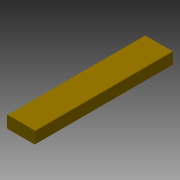
# Autodesk Inventor part: 2x4x17
Saved by Autodesk Inventor 2015 (Build 190159000, 159)
## iProperties
Created: 2015-01-03
Part Number: 2x4x17
Material: Wood (Oak)
Document SubType Name: Modeling
Designer: Peter
Mass: 3130.43 g
Surface Area: 3097.88 cm^2
Volume: 4118.99 cm^3
Density: 0.76 g/cm^3
Appearance: Gold
Author: Peter
Autodesk Inventor part; units mm, degrees
ref_plane "YZ Plane" through (0, 0, 0) normal (1, 0, 0) x (0, 1, 0)
ref_plane "XZ Plane" through (0, 0, 0) normal (0, 1, 0) x (-1, 0, 0)
ref_plane "XY Plane" through (0, 0, 0) normal (0, 0, 1) x (1, 0, 0)
sketch "Sketch1" plane through (0, 0, 0) normal (0, 0, 1) x (1, 0, 0)
  line L0 (0, 0) -> (88.9, 0)
  line L1 (88.9, 0) -> (88.9, 34.925)
  line L2 (85.725, 38.1) -> (3.175, 38.1)
  line L3 (0, 34.925) -> (0, 0)
  arc A0 (3.175, 38.1) -> (0, 34.925) centre (3.175, 34.925) ccw
  arc A1 (88.9, 34.925) -> (85.725, 38.1) centre (85.725, 34.925) ccw
  point P0 (88.9, 38.1)
  point P1 (0, 38.1)
  dimension "Width" = 88.9
  dimension "Height" = 38.1
  dimension "d2" = 3.175
  constraints: 8 end point, 4 point on circle, 4 point on line, 4 tangent, 2 centre point, 2 parallel, 1 equal radius, 1 horizontal, 1 perpendicular
  measures "Width" distance of point (88.9, 38.1) point (0, 38.1)
  measures "Height" distance of L0.end point (88.9, 38.1)
  measures "d2" radius of A0
extrude "Extrusion1" add sketch "Sketch1" along normal blind 431.8
fillet "Fillet1" radius 3.175 1 edges at (88.9, 0, 215.9)
fillet "Fillet2" radius 3.175 1 edges at (0, 0, 215.9)
body "Solid1"
